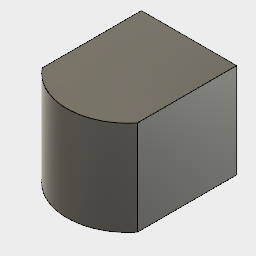
simplified_body (Autodesk Fusion 360 design; units mm, degrees)
Autodesk Fusion 360 part; units mm, degrees
sketch "Sketch1" plane through (0, 0, 0) normal (0, 1, 0) x (1, 0, 0)
sketch "Sketch2" plane through (0, 0, 0) normal (0, 1, 0) x (1, 0, 0)
sketch "Sketch3" plane through (0, 0, 0) normal (0, 1, 0) x (1, 0, 0)
  line L0 (46.8, 60) -> (46.8, -60) construction
  line L1 (46.8, -60) -> (-46.8, -60) construction
  line L2 (-46.8, -60) -> (-46.8, 60) construction
  line L3 (-46.8, 60) -> (46.8, 60) construction
  line L4 (0, 70) -> (0, -70) construction
  arc A0 (-46.8, -37.5468) -> (46.8, -37.5468) centre (0, 0) ccw
  line L5 (-46.8, -37.5468) -> (-46.8, 60)
  line L6 (-46.8, 60) -> (46.8, 60)
  line L7 (46.8, 60) -> (46.8, -37.5468)
  dimension "d1" = 120
  dimension "d2" = 60
  dimension "d3" = 46.8
  dimension "d4" = 60
  constraint vertical L0
  constraint perpendicular L0 L1
  constraint perpendicular L1 L2
  constraint perpendicular L0 L3
  constraint perpendicular L3 L4
  constraint coincident L0 A0.centre
  constraint coincident L2 A0.centre
  constraint coincident A0.centre origin
extrude "Extrude1" add sketch "Sketch3" along normal blind 93
